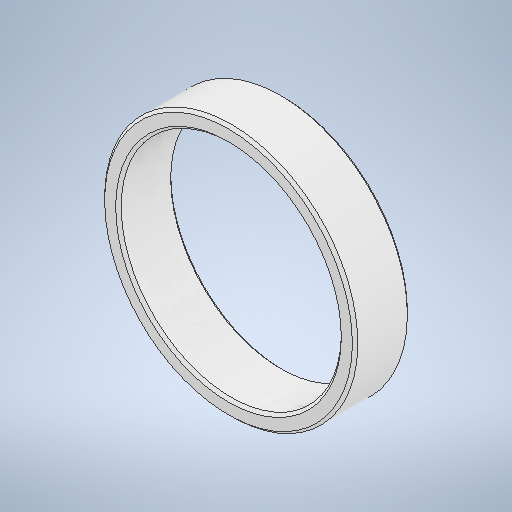
# Autodesk Inventor part: 35-30-xxx Plain Bearing Socket
Saved by Autodesk Inventor 2025 (Build 290162000, 162)
## iProperties
Created: 2025-01-03
Part Number: 35-30-xxx Plain Bearing Socket
Material: Kunststoff, undurchsichtig Weiß
Document SubType Name: Modeling
Designer: marco.benkert
Density: 0.952 g/cm^3
Appearance: Glatt - Weiß
Author: marco.benkert
Autodesk Inventor part; units mm, degrees
ref_plane "YZ Plane" through (0, 0, 0) normal (1, 0, 0) x (0, 1, 0)
ref_plane "XZ Plane" through (0, 0, 0) normal (0, 1, 0) x (-1, 0, 0)
ref_plane "XY Plane" through (0, 0, 0) normal (0, 0, 1) x (1, 0, 0)
sketch "Skizze1" plane through (0, 0, 0) normal (1, 0, 0) x (0, 1, 0)
  line L0 (5, 23) -> (-5, 23)
  line L1 (-5, 23) -> (-5, 20)
  line L2 (-5, 20) -> (5, 20)
  line L3 (5, 20) -> (5, 23)
  line L4 (5.4713, 0) -> (-6.5925, 0)
  point P0 (0, 0)
  point P1 (0, 20)
  point P2 (0, 23)
  dimension "d0" = 20
  dimension "d1" = 23
  dimension "d2" = 10
  dimension "d3" = 5
  constraints: 10 end point, 2 horizontal, 2 midpoint, 2 parallel, 1 perpendicular
  measures "d0" distance of point (0, 0) point (0, 20)
  measures "d1" distance of point (0, 23) point (0, 0)
  measures "d2" distance of L0.end L0.start
  measures "d3" distance from line of point (0, 0) L1
revolve "Basebody" add sketch "Skizze1" angle 360 about axis through (0, 5.4713, 0) along (0, -1, 0)
chamfer "Fasen1" distance 0.5 angle 45 4 edges at (0, 5, -20) (0, 5, -23) (0, -5, -23) (0, -5, -20)
